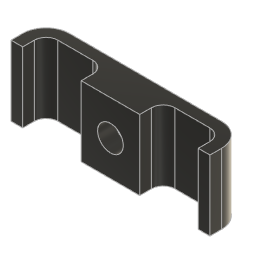
cable-clip (Autodesk Fusion 360 design; units mm, degrees)
Autodesk Fusion 360 part; units mm, degrees
sketch "Sketch1" plane through (0, 0, 0) normal (0, 0, 1) x (1, 0, 0)
  line L0 (-2.5, 0) -> (-2.5, 1)
  line L1 (-3.5, 2) -> (-6.5, 2)
  line L2 (-7.5, 1) -> (-7.5, 0)
  line L3 (0, 0) -> (-2.5, 0)
  line L4 (-7.5, 0) -> (-8.5, 0)
  line L5 (-8.5, 0) -> (-8.5, 1)
  line L6 (-6.5, 3) -> (0, 3)
  arc A0 (-6.5, 2) -> (-7.5, 1) centre (-6.5, 1) ccw
  arc A1 (-2.5, 1) -> (-3.5, 2) centre (-3.5, 1) ccw
  arc A2 (-6.5, 3) -> (-8.5, 1) centre (-6.5, 1) ccw
  line L7 (0, 0) -> (0, 3) construction
  line L8 (0, 0) -> (2.5, 0)
  line L9 (2.5, 0) -> (2.5, 1)
  arc A3 (3.5, 2) -> (2.5, 1) centre (3.5, 1) ccw
  line L10 (3.5, 2) -> (6.5, 2)
  arc A4 (7.5, 1) -> (6.5, 2) centre (6.5, 1) ccw
  line L11 (7.5, 1) -> (7.5, 0)
  line L12 (7.5, 0) -> (8.5, 0)
  line L13 (8.5, 0) -> (8.5, 1)
  arc A5 (8.5, 1) -> (6.5, 3) centre (6.5, 1) ccw
  line L14 (6.5, 3) -> (0, 3)
  dimension "d1" = 1
  dimension "d2" = 2
  dimension "d3" = 5
  dimension "d4" = 1
  dimension "d5" = 1
  dimension "d8" = 5
  constraint perpendicular L0 L1
  constraint coincident L3.start L7.start
  constraint perpendicular L0 L3
  constraint perpendicular L2 L4
  constraint perpendicular L1 L5
  constraint perpendicular L5 L6
  constraint tangent L1 A0
  constraint tangent L2 A0
  constraint tangent L0 A1
  constraint tangent L1 A1
  constraint equal A0 A1
  constraint tangent L5 A2
  constraint tangent L6 A2
  constraint horizontal L3
  constraint coincident A0.centre A2.centre
  constraint collinear L3 L4
  constraint perpendicular L3 L7
  constraint coincident L6.end L7.end
  constraint symmetric L0.start L7 L8.end
  constraint symmetric L2.end L7 L11.end
  constraint symmetric L3.start L7 L8.start
  constraint symmetric L4.end L7 L12.end
  constraint symmetric L6.end L7 L14.end
  constraint symmetric L1.end L7 L10.end
  constraint symmetric L2.start L7 A4.start
  constraint symmetric A0 L7 A4
  constraint symmetric L0.end L7 L9.end
  constraint symmetric L1.start L7 A3.start
  constraint symmetric A1 L7 A3
  constraint symmetric L5.end L7 L13.end
  constraint symmetric L6.start L7 A5.end
  constraint symmetric A2 L7 A5
  measures "d1" radius of A0
  measures "d2" distance of L1 L3
  measures "d3" distance of L0 L2
  measures "d4" distance of L1 L6
  measures "d5" distance of L2 L5
  measures "d8" distance of L0 L9
extrude "Extrude1" add sketch "Sketch1" along normal blind 6
sketch "Sketch4" plane through (0, 3, 0) normal (0, 1, 0) x (-1, 0, 0)
  line L0 (-6.5, 0) -> (6.5, 0) construction
  line L1 (6.5, 0) -> (6.5, 6) construction
  line L2 (6.5, 6) -> (-6.5, 6) construction
  line L3 (-6.5, 6) -> (-6.5, 0) construction
  line L4 (-6.5, 6) -> (6.5, 0) construction
  circle A0 centre (0, 3) radius 1.75
  dimension "d11" = 3.5
  constraint coincident L2.end L3.start
  constraint coincident L0.end L1.start
  constraint midpoint L4 A0.centre
  measures "d11" diameter of A0
hole "Hole1" at (0, 3, 3) direction (0, -1, 0) diameter 2.2 end through all counterbore diameter 3.5 counterbore depth 1.5
